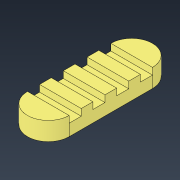
# Autodesk Inventor part: Dribblerdaempfer Unten
Saved by Autodesk Inventor 2022.1 (Build 261234020, 234B)
## iProperties
Part Number: Dribblerdaempfer Unten
Material: Gummi, Silikon
Document SubType Name: Modeling
Designer: rYan
Density: 1.25 g/cm^3
Appearance: Gummi - Schwarz
Mass: 0.162496 g
Surface Area: 2.40547 cm^2
Volume: 0.129997 cm^3
Author: rYan
Autodesk Inventor part; units mm, degrees
ref_plane "YZ Plane" through (0, 0, 0) normal (1, 0, 0) x (0, 1, 0)
ref_plane "XZ Plane" through (0, 0, 0) normal (0, 1, 0) x (-1, 0, 0)
ref_plane "XY Plane" through (0, 0, 0) normal (0, 0, 1) x (1, 0, 0)
sketch "Skizze1" plane through (0, 0, 0) normal (0, 0, 1) x (1, 0, 0)
  line L0 (0, -5) -> (0, 5) construction
  line L1 (2.5, -5) -> (2.5, 5)
  line L2 (-2.5, 5) -> (-2.5, -5)
  arc A0 (-2.5, -5) -> (2.5, -5) centre (0, -5) ccw
  arc A1 (2.5, 5) -> (-2.5, 5) centre (0, 5) ccw
  point P0 (0, 0)
  dimension "d0" = 5
  dimension "d1" = 10
  constraints: 8 end point, 4 point on circle, 4 tangent, 2 centre point, 1 midpoint, 1 parallel, 1 vertical
  measures "d0" diameter of A1
  measures "d1" distance of L0.start L0.end
extrude "Extrusion1" add sketch "Skizze1" along normal blind 1.4
sketch "Skizze2" plane through (0, 0, 1.4) normal (0, 0, 1) x (1, 0, 0)
  line L0 (2.5, -5) -> (2.5, 5) projected
  arc A0 (2.5, 5) -> (-2.5, 5) centre (0, 5) ccw projected
  line L1 (-2.5, 5) -> (-2.5, -5) projected
  arc A1 (-2.5, -5) -> (2.5, -5) centre (0, -5) ccw projected
  line L2 (-2.5, 5) -> (-2.5, -5) projected
  line L3 (-2.5, 5) -> (2.5, 5)
  line L4 (2.5, -5) -> (2.5, 5) projected
  line L5 (2.5, -5) -> (-2.5, -5)
  arc A2 (2.5, 5) -> (-2.5, 5) centre (0, 5) ccw
  arc A3 (-2.5, -5) -> (2.5, -5) centre (0, -5) ccw
  line L6 (-2.5, 3.55) -> (2.5, 3.55)
  line L7 (2.5, 3.55) -> (2.5, 2.15)
  line L8 (2.5, 2.15) -> (-2.5, 2.15)
  line L9 (-2.5, 2.15) -> (-2.5, 3.55)
  line L10 (2.5, 0.7) -> (-2.5, 0.7)
  line L11 (-2.5, 0.7) -> (-2.5, -0.7)
  line L12 (-2.5, -0.7) -> (2.5, -0.7)
  line L13 (2.5, -0.7) -> (2.5, 0.7)
  line L14 (-2.5, -2.15) -> (2.5, -2.15)
  line L15 (2.5, -2.15) -> (2.5, -3.55)
  line L16 (2.5, -3.55) -> (-2.5, -3.55)
  line L17 (-2.5, -3.55) -> (-2.5, -2.15)
  line L18 (-3.5, 0) -> (3.5, 0) projected
  line L19 (-2.5, 2.85) -> (2.5, 2.85) construction
  point P0 (0, 0)
  dimension "d4" = 1.4
  dimension "d5" = 1.4
  constraints: 30 end point, 6 parallel, 6 point on line, 5 perpendicular, 4 point on circle, 4 tangent, 3 horizontal, 2 centre point, 2 midpoint, 4 other
  measures "d4" distance of L10.end L11.end
  measures "d5" distance of L8.end L6.start
extrude "Extrusion2" add sketch "Skizze2" along normal blind 0.8 contours A1 L5 | L16 L1 L14 L0 | L12 L1 L18 L0 | L18 L1 L10 L0 | L8 L1 L6 L0 | L3 A0
equation "\"d5\" = d4"
